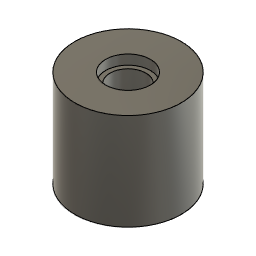
Gehaeuse (Autodesk Fusion 360 archive; units mm, degrees)
design "Befestigungsrohr"
Autodesk Fusion 360 part; units mm, degrees
sketch "Skizze1" plane through (0, 0, 0) normal (0, 1, 0) x (1, 0, 0)
sketch "Skizze2" plane through (0, 0, 0) normal (0, 1, 0) x (1, 0, 0)
  circle A0 centre (-32.0905, 19.022) radius 2.75
  circle A1 centre (-32.0905, 19.022) radius 0.925
  dimension "d1" = 5.5
  dimension "d2" = 1.85
  constraint concentric A0 A1
  measures "d1" diameter of A0
  measures "d2" diameter of A1
extrude "Extrusion1" add sketch "Skizze2" along normal blind 5
sketch "Skizze3" plane through (0, 5, 0) normal (0, 1, 0) x (-1, 0, 0)
  circle A0 centre (32.0905, -19.022) radius 0.925
  circle A1 centre (32.0905, -19.022) radius 2.75
  circle A2 centre (32.0905, -19.022) radius 1.155
  dimension "d5" = 2.31
  constraint concentric A0 A2
  measures "d5" diameter of A2
extrude "Extrusion2" cut sketch "Skizze3" against normal blind 0.5 contours A2

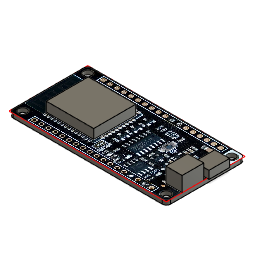
design "Microcontroller"
Autodesk Fusion 360 part; units mm, degrees
sketch "Skizze1" plane through (0, 0, 0) normal (0, 1, 0) x (1, 0, 0)
  line L0 (-42.4258, 18.0352) -> (12.5742, 18.0352)
  line L1 (14.0742, 16.5352) -> (14.0742, -9.4648)
  line L2 (12.5742, -10.9648) -> (-42.4258, -10.9648)
  line L3 (-43.9258, -9.4648) -> (-43.9258, 16.5352)
  line L4 (-14.9258, 20.3575) -> (-14.9258, -19.985) construction
  line L5 (-54.1584, 3.5352) -> (25.7033, 3.5352) construction
  circle A0 centre (-41.4258, 15.5352) radius 1.5
  circle A1 centre (11.5742, 15.5352) radius 1.5
  circle A2 centre (-41.4258, -8.4648) radius 1.5
  circle A3 centre (11.5742, -8.4648) radius 1.5
  arc A4 (-42.4258, 18.0352) -> (-43.9258, 16.5352) centre (-42.4258, 16.5352) ccw
  arc A5 (-43.9258, -9.4648) -> (-42.4258, -10.9648) centre (-42.4258, -9.4648) ccw
  arc A6 (12.5742, -10.9648) -> (14.0742, -9.4648) centre (12.5742, -9.4648) ccw
  arc A7 (14.0742, 16.5352) -> (12.5742, 18.0352) centre (12.5742, 16.5352) ccw
  line L6 (-36.7258, 11.0352) -> (-19.2258, 11.0352)
  line L7 (-19.2258, 11.0352) -> (-19.2258, -4.4648)
  line L8 (-19.2258, -4.4648) -> (-36.7258, -4.4648)
  line L9 (-36.7258, -4.4648) -> (-36.7258, 11.0352)
  line L10 (14.7742, 11.6352) -> (9.2742, 11.6352)
  line L11 (9.2742, 11.6352) -> (9.2742, 4.0352)
  line L12 (9.2742, 4.0352) -> (14.7742, 4.0352)
  line L13 (14.7742, 4.0352) -> (14.7742, 11.6352)
  line L14 (8.0742, 2.8352) -> (14.0742, 2.8352)
  line L15 (14.0742, 2.8352) -> (14.0742, -5.1648)
  line L16 (14.0742, -5.1648) -> (8.0742, -5.1648)
  line L17 (8.0742, -5.1648) -> (8.0742, 2.8352)
  point P0 (-43.9258, 18.0352)
  point P1 (14.0742, 18.0352)
  point P2 (-43.9258, -10.9648)
  dimension "d1" = 58
  dimension "d2" = 29
  dimension "d3" = 3
  dimension "d4" = 26.5
  dimension "d5" = 12
  dimension "d6" = 1.5
  dimension "d9" = 17.5
  dimension "d10" = 15.5
  dimension "d11" = 6.5
  dimension "d12" = 7.2
  dimension "d15" = 5.5
  dimension "d16" = 7.6
  dimension "d17" = 0.7
  dimension "d18" = 6.4
  dimension "d23" = 8
  dimension "d24" = 6
  dimension "d26" = 5.8
  constraint horizontal L0
  constraint vertical L1
  constraint horizontal L2
  constraint vertical L3
  constraint perpendicular L2 L4
  constraint symmetric L1 L3 L4
  constraint perpendicular L3 L5
  constraint symmetric L0 L2 L5
  constraint symmetric L4 A0 A1
  constraint symmetric L5 A0 A2
  constraint symmetric L5 A1 A3
  constraint coincident P0 L0
  constraint coincident P0 L3
  constraint tangent L0 A4
  constraint tangent L3 A4
  constraint coincident P2 L2
  constraint coincident P2 L3
  constraint tangent L2 A5
  constraint tangent L3 A5
  constraint equal A4 A5
  constraint tangent L1 A6
  constraint tangent L2 A6
  constraint equal A4 A6
  constraint coincident P1 L0
  constraint coincident P1 L1
  constraint tangent L0 A7
  constraint tangent L1 A7
  constraint equal A4 A7
  constraint horizontal L6
  constraint vertical L7
  constraint horizontal L8
  constraint vertical L9
  constraint horizontal L10
  constraint vertical L11
  constraint horizontal L12
  constraint vertical L13
  constraint horizontal L14
  constraint vertical L15
  constraint horizontal L16
  constraint vertical L17
  constraint coincident L1 L15.end
  measures "d1" distance of P0 P1
  measures "d2" distance of P0 P2
  measures "d3" diameter of A0
  measures "d4" distance of L4 A0.centre
  measures "d5" distance of L5 A0.centre
  measures "d6" radius of A4
  measures "d9" distance of L7.end L8.end
  measures "d10" distance of L6.end L7.end
  measures "d11" distance of L2 L8
  measures "d12" distance of L3 L9
  measures "d15" distance of L10.start L10.end
  measures "d16" distance of L10.end L11.end
  measures "d17" distance of L1 L13
  measures "d18" distance of L0 L10
  measures "d23" distance of L14.start L16.end
  measures "d24" distance of L14.start L14.end
  measures "d26" distance of L2 L16
extrude "Extrusion1" add sketch "Skizze1" along normal blind 1.5 contours L0 L1 L2 L3 A4 A5 A6 A7 L10 L11 L12 L14 L16 L17 | L1 L10 L11 L12 | L1 L14 L15 L16 L17 | L6 L7 L8 L9
extrude "Extrusion2" add sketch "Skizze1" along normal blind 5 contours L6 L7 L8 L9
extrude "Extrusion3" add sketch "Skizze1" along normal blind 4.4 and the other way blind -1.5 contours L1 L10 L12 L13 | L1 L10 L11 L12
extrude "Extrusion4" add sketch "Skizze1" along normal blind 7 contours L1 L14 L15 L16 L17
equation "d4 = ( 53 / 2 ) * 1 mm"
equation "d5 = ( 24 / 2 ) * 1 mm"

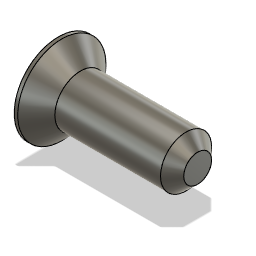
design "Schraube"
Autodesk Fusion 360 part; units mm, degrees
sketch "Skizze1" plane through (0, 0, 0) normal (0, 1, 0) x (1, 0, 0)
  line L0 (-39.2641, 12.0215) -> (10.8095, 12.0215) construction
  line L1 (-30.9471, 12.0215) -> (-30.9471, 13.9215)
  line L2 (-30.9471, 13.9215) -> (-30.7971, 13.9215)
  line L3 (-30.7971, 13.9215) -> (-29.9971, 13.1215)
  line L4 (-29.9971, 13.1215) -> (-24.9471, 13.1215)
  line L5 (-24.9471, 13.1215) -> (-24.9471, 12.0215)
  line L6 (-30.9471, 12.0215) -> (-24.9471, 12.0215)
  dimension "d1" = 135
  dimension "d2" = 6
  dimension "d3" = 1.1
  dimension "d4" = 1.9
  dimension "d5" = 0.15
  constraint horizontal L0
  constraint coincident L0 L1.start
  constraint perpendicular L0 L1
  constraint perpendicular L1 L2
  constraint perpendicular L1 L4
  constraint coincident L0 L5.end
  constraint perpendicular L0 L5
  measures "d1" angle of L3 L4
  measures "d2" distance of L1 L5
  measures "d3" distance of L4 L5.end
  measures "d4" distance of L0 L2
  measures "d5" distance of L1.end L2.end
revolve "Drehen1" add sketch "Skizze1" angle 360 about axis through (-39.2641, 0, -12.0215) along (1, 0, 0)
chamfer "Fase1" distance 0.5 angle 45 1 edges at (-24.9471, -0.3978, -10.9959)
sketch "Skizze2" plane through (-30.9471, 0, 0) normal (-1, 0, 0) x (0, 0, 1)
  circle A0 centre (-12.0215, 0) radius 1.9
  circle A1 centre (-12.0215, 0) radius 0.875
  dimension "d8" = 1.75
  constraint concentric A0 A1
  measures "d8" diameter of A1
extrude "Extrusion1" cut sketch "Skizze2" against normal blind 0.8 contours A1
equation "d4 = ( 3.8 / 2 ) * 1 mm"

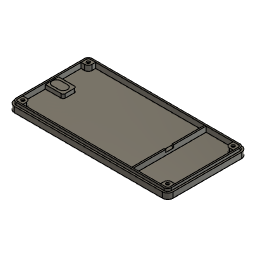
design "Gehäuseboden"
Autodesk Fusion 360 part; units mm, degrees
sketch "Skizze1" plane through (0, 0, 0) normal (0, 1, 0) x (1, 0, 0)
  line L0 (-57.1853, 33.6695) -> (54.8147, 33.6695)
  line L1 (58.8147, 29.6695) -> (58.8147, -22.3305)
  line L2 (54.8147, -26.3305) -> (-57.1853, -26.3305)
  line L3 (-61.1853, -22.3305) -> (-61.1853, 29.6695)
  arc A0 (-57.1853, 33.6695) -> (-61.1853, 29.6695) centre (-57.1853, 29.6695) ccw
  arc A1 (-61.1853, -22.3305) -> (-57.1853, -26.3305) centre (-57.1853, -22.3305) ccw
  arc A2 (54.8147, -26.3305) -> (58.8147, -22.3305) centre (54.8147, -22.3305) ccw
  arc A3 (58.8147, 29.6695) -> (54.8147, 33.6695) centre (54.8147, 29.6695) ccw
  point P0 (-61.1853, 33.6695)
  point P1 (58.8147, 33.6695)
  point P2 (-61.1853, -26.3305)
  dimension "d1" = 120
  dimension "d2" = 60
  dimension "d3" = 4
  constraint horizontal L0
  constraint vertical L1
  constraint horizontal L2
  constraint vertical L3
  constraint coincident P0 L0
  constraint coincident P0 L3
  constraint tangent L0 A0
  constraint tangent L3 A0
  constraint coincident P2 L2
  constraint coincident P2 L3
  constraint tangent L2 A1
  constraint tangent L3 A1
  constraint equal A0 A1
  constraint tangent L1 A2
  constraint tangent L2 A2
  constraint equal A0 A2
  constraint coincident P1 L0
  constraint coincident P1 L1
  constraint tangent L0 A3
  constraint tangent L1 A3
  constraint equal A0 A3
  measures "d1" distance of P0 P1
  measures "d2" distance of P0 P2
  measures "d3" radius of A0
extrude "Extrusion1" add sketch "Skizze1" against normal blind 2.5 makes body 1
ref_plane "Arbeitsebene1" through (-1.1853, -1.25, -3.6695) normal (1, 0, 0) x (0, 0, 1)
sketch "Skizze4" plane through (-1.1853, -1.25, -3.6695) normal (1, 0, 0) x (0, 0, -1)
  line L0 (-27.5, 5.25) -> (-28.65, 5.25)
  line L1 (-28.65, 5.25) -> (-28.65, 3.25)
  line L2 (-28.65, 3.25) -> (-30, 3.25)
  line L3 (-30, 3.25) -> (-30, 1.25)
  line L4 (-30, 1.25) -> (-27.5, 1.25)
  line L5 (-27.5, 5.25) -> (-27.5, 1.25)
  line L6 (26, 1.25) -> (-26, 1.25)
  dimension "d16" = 1.5
  dimension "d17" = 2.5
  dimension "d18" = 1.15
  dimension "d28" = 4
  dimension "d29" = 2
  constraint horizontal L0
  constraint perpendicular L0 L1
  constraint perpendicular L1 L2
  constraint perpendicular L2 L3
  constraint perpendicular L3 L4
  constraint perpendicular L4 L5
  constraint collinear L4 L6
  measures "d16" distance of L5 L6.end
  measures "d17" distance of L3.end L4.end
  measures "d18" distance of L0.start L0.end
  measures "d28" distance of L0.start L4.end
  measures "d29" distance of L0.end L1.end
sweep "Sweeping1" add profiles "Skizze4" along 8 edges at (-60.0137, 0, 25.1589) (-61.1853, 0, -3.6695) (-60.0137, 0, -32.4979) (-1.1853, 0, -33.6695) (57.6431, 0, -32.4979) (58.8147, 0, -3.6695) (57.6431, 0, 25.1589) (-1.1853, 0, 26.3305) section 1 on bodies 1 bodies 1
ref_plane "Arbeitsebene2" through (-1.1853, -0.25, -3.6695) normal (0, 0, 1) x (-1, 0, 0)
sketch "Skizze5" plane through (-1.1853, -0.25, -3.6695) normal (0, 0, 1) x (1, 0, 0)
  line L0 (29, 0.25, -27.5) -> (31.5, 0.25, -27.5)
  line L1 (31.5, 0.25, -27.5) -> (31.5, 4.25, -27.5)
  line L2 (31.5, 4.25, -27.5) -> (30.35, 4.25, -27.5)
  line L3 (30.35, 4.25, -27.5) -> (30.35, 2.25, -27.5)
  line L4 (30.35, 2.25, -27.5) -> (29, 2.25, -27.5)
  line L5 (29, 2.25, -27.5) -> (29, 0.25, -27.5)
  line L6 (56, 0.25, -27.5) -> (-56, 0.25, -27.5)
  line L7 (56, 4.25, -27.5) -> (56, 0.25, -27.5)
  dimension "d35" = 2.5
  dimension "d36" = 4
  dimension "d37" = 2
  dimension "d38" = 1.15
  dimension "d39" = 24.5
extrude "Extrusion2" add sketch "Skizze5" along normal up to near side of body 1 separate body contours L0 L1 L2 L3 L4 L5 L6 in plane through (-1.1853, -0.25, -31.1695) normal (0, 0, 1) makes body 2
sketch "Skizze6" plane through (30.3147, 0, 0) normal (1, 0, 0) x (0, 0, -1)
  line L0 (-23.8305, 4) -> (-23.8305, 0)
  line L1 (-23.8305, 0) -> (31.1695, 0)
  line L2 (31.1695, 0) -> (31.1695, 4)
  line L3 (31.1695, 4) -> (-23.8305, 4)
sketch "Skizze7" plane through (30.3147, 2, -3.6695) normal (1, 0, 0) x (0, 0, -1)
  line L0 (3, 2) -> (3, 0)
  line L1 (3, 0) -> (-3, 0)
  line L2 (-3, 0) -> (-3, 2)
  line L3 (27.5, 2) -> (-27.5, 2)
  line L4 (27.5, -2) -> (27.5, 2)
  line L5 (-27.5, 2) -> (-27.5, -2)
  line L6 (-3, 2) -> (3, 2)
  dimension "d42" = 6
  dimension "d43" = 2
  dimension "d44" = 24.5
  dimension "d45" = 24
  constraint vertical L0
  constraint perpendicular L0 L1
  constraint perpendicular L1 L2
  constraint coincident L3 L2.end
  constraint coincident L3 L0.start
  measures "d42" distance of L0.end L1.end
  measures "d43" distance of L1 L3
  measures "d44" distance of L0 L4
extrude "Extrusion3" cut sketch "Skizze7" against normal blind 3 bodies 2
chamfer "Fase1" distance 0.3 angle 45 1 faces at (17.4814, -2.5, 6.3305) on bodies 1
sketch "Skizze8" plane through (0, 0, 0) normal (0, 1, 0) x (-1, 0, 0)
  arc A0 (-54.8147, 23.8305) -> (-56.3147, 22.3305) centre (-54.8147, 22.3305) ccw
  line L0 (-56.3147, 22.3305) -> (-56.3147, -29.6695)
  arc A1 (-56.3147, -29.6695) -> (-54.8147, -31.1695) centre (-54.8147, -29.6695) ccw
  line L1 (-54.8147, -31.1695) -> (57.1853, -31.1695)
  arc A2 (57.1853, -31.1695) -> (58.6853, -29.6695) centre (57.1853, -29.6695) ccw
  line L2 (58.6853, -29.6695) -> (58.6853, 22.3305)
  arc A3 (58.6853, 22.3305) -> (57.1853, 23.8305) centre (57.1853, 22.3305) ccw
  line L3 (57.1853, 23.8305) -> (-54.8147, 23.8305)
  line L4 (58.6853, 18.3305) -> (55.9353, 18.3305)
  line L5 (53.1853, 21.0805) -> (53.1853, 23.8305)
  line L6 (53.1853, 23.8305) -> (58.6853, 23.8305)
  line L7 (58.6853, 23.8305) -> (58.6853, 18.3305)
  arc A4 (53.1853, 21.0805) -> (55.9353, 18.3305) centre (55.9353, 21.0805) ccw
  line L8 (-50.8147, -31.1695) -> (-56.3147, -31.1695)
  line L9 (-56.3147, -31.1695) -> (-56.3147, -25.6695)
  line L10 (-56.3147, -25.6695) -> (-53.5647, -25.6695)
  line L11 (-50.8147, -28.4195) -> (-50.8147, -31.1695)
  arc A5 (-50.8147, -28.4195) -> (-53.5647, -25.6695) centre (-53.5647, -28.4195) ccw
  point P0 (53.1853, 18.3305)
  point P1 (-50.8147, -25.6695)
  dimension "d49" = 5.5
  dimension "d50" = 5.5
  dimension "d51" = 2.75
  dimension "d52" = 5.5
  dimension "d53" = 5.5
  dimension "d54" = 2.75
  constraint horizontal L4
  constraint vertical L5
  constraint horizontal L6
  constraint vertical L7
  constraint coincident L3 L5.end
  constraint coincident L2 L4.start
  constraint coincident P0 L4
  constraint coincident P0 L5
  constraint tangent L4 A4
  constraint tangent L5 A4
  constraint horizontal L8
  constraint vertical L9
  constraint horizontal L10
  constraint vertical L11
  constraint coincident L0 L9.end
  constraint coincident L1 L8.start
  constraint coincident P1 L10
  constraint coincident P1 L11
  constraint tangent L10 A5
  constraint tangent L11 A5
  measures "d49" distance of L4.start P0
  measures "d50" distance of P0 L5.end
  measures "d51" radius of A4
  measures "d52" distance of L9.end P1
  measures "d53" distance of L8.start P1
  measures "d54" radius of A5
extrude "Extrusion4" add sketch "Skizze8" along normal up to surface (4 mm away) separate body contours L2 A3 L3 L4 L5 L6 L7 A4 | L0 A1 L1 L8 L9 L10 L11 A5 makes body 3 at (-55.9353, 0, 20.5805) makes body 4 at (53.0647, 0, -28.4195)
sketch "Skizze9" plane through (0, 4, 0) normal (0, 1, 0) x (-1, 0, 0)
  line L0 (57.1853, 23.8305) -> (53.1853, 23.8305)
  line L1 (53.1853, 23.8305) -> (53.1853, 21.0805)
  arc A0 (53.1853, 21.0805) -> (55.9353, 18.3305) centre (55.9353, 21.0805) ccw
  line L2 (55.9353, 18.3305) -> (58.6853, 18.3305)
  line L3 (58.6853, 18.3305) -> (58.6853, 22.3305)
  arc A1 (58.6853, 22.3305) -> (57.1853, 23.8305) centre (57.1853, 22.3305) ccw
  circle A2 centre (55.9353, 21.0805) radius 1.225
  circle A3 centre (-53.5647, -28.4195) radius 1.225
  line L4 (-50.8147, -28.4195) -> (-50.8147, -31.1695)
  point P0 (-53.5647, -25.6695)
  dimension "d57" = 2.45
  dimension "d58" = 2.45
  dimension "d59" = 2.75
  dimension "d60" = 2.75
  constraint concentric A0 A2
  measures "d57" diameter of A2
  measures "d58" diameter of A3
  measures "d59" distance of A3.centre L4
  measures "d60" distance of A3.centre P0
extrude "Extrusion5" cut sketch "Skizze9" against normal up to surface (6.5 mm away) contours A2 | A3 bodies 1 3 4
sketch "Skizze10" plane through (0, -2.5, 0) normal (0, -1, 0) x (1, 0, 0)
  circle A0 centre (-55.9353, 21.0805) radius 1.225
  circle A1 centre (53.5647, -28.4195) radius 1.225
  arc A2 (58.5147, 22.3305) -> (54.8147, 26.0305) centre (54.8147, 22.3305) ccw
  line L0 (54.8147, 26.0305) -> (-57.1853, 26.0305)
  arc A3 (-57.1853, 26.0305) -> (-60.8853, 22.3305) centre (-57.1853, 22.3305) ccw
  line L1 (-60.8853, 22.3305) -> (-60.8853, -29.6695)
  arc A4 (-60.8853, -29.6695) -> (-57.1853, -33.3695) centre (-57.1853, -29.6695) ccw
  line L2 (-57.1853, -33.3695) -> (54.8147, -33.3695)
  arc A5 (54.8147, -33.3695) -> (58.5147, -29.6695) centre (54.8147, -29.6695) ccw
  line L3 (58.5147, -29.6695) -> (58.5147, 22.3305)
  circle A6 centre (-55.9353, 21.0805) radius 2.25
  circle A7 centre (53.5647, -28.4195) radius 2.25
  circle A8 centre (-55.9353, -28.4195) radius 2.25
  circle A9 centre (53.5647, 21.0805) radius 2.25
  line L4 (-58.6853, 22.3305) -> (-58.6853, -29.6695)
  line L5 (-57.1853, -31.1695) -> (54.8147, -31.1695)
  line L6 (56.3147, -29.6695) -> (56.3147, 22.3305)
  line L7 (54.8147, 23.8305) -> (-57.1853, 23.8305)
  dimension "d63" = 4.5
  dimension "d64" = 4.5
  dimension "d93" = 4.5
  dimension "d94" = 4.5
  dimension "d95" = 2.75
  dimension "d96" = 2.75
  dimension "d97" = 2.75
  dimension "d98" = 2.75
  constraint concentric A0 A6
  constraint concentric A1 A7
  measures "d63" diameter of A6
  measures "d64" diameter of A7
  measures "d93" diameter of A8
  measures "d94" diameter of A9
  measures "d95" distance of A8.centre L4
  measures "d96" distance of A8.centre L5
  measures "d97" distance of A9.centre L6
  measures "d98" distance of A9.centre L7
extrude "Extrusion6" cut sketch "Skizze10" against normal blind 4.5 contours A6 | A7 bodies 1 3 4
chamfer "Fase2" distance 1 angle 45 2 edges at (-54.7932, 2, 21.5235) (54.7068, 2, -27.9765) on bodies 3 4
chamfer "Fase3" distance 0.15 angle 45 2 edges at (-58.0331, -2.5, 21.8941) (51.4669, -2.5, -27.6059) on bodies 1
sketch "Skizze11" plane through (0, 0, 0) normal (0, 1, 0) x (-1, 0, 0)
  circle A0 centre (55.9353, 21.0805) radius 2.25
  circle A1 centre (-53.5647, -28.4195) radius 2.25
  arc A2 (-54.8147, 23.8305) -> (-56.3147, 22.3305) centre (-54.8147, 22.3305) ccw
  line L0 (-56.3147, 22.3305) -> (-56.3147, -29.6695)
  arc A3 (-56.3147, -29.6695) -> (-54.8147, -31.1695) centre (-54.8147, -29.6695) ccw
  line L1 (-54.8147, -31.1695) -> (57.1853, -31.1695)
  arc A4 (57.1853, -31.1695) -> (58.6853, -29.6695) centre (57.1853, -29.6695) ccw
  line L2 (58.6853, -29.6695) -> (58.6853, 22.3305)
  arc A5 (58.6853, 22.3305) -> (57.1853, 23.8305) centre (57.1853, 22.3305) ccw
  line L3 (57.1853, 23.8305) -> (-54.8147, 23.8305)
  line L4 (55.1853, -5.4195) -> (52.9239, -5.4195)
  line L5 (55.1853, -1.9195) -> (52.9239, -1.9195)
  arc A6 (55.1853, -5.4195) -> (55.1853, -1.9195) centre (55.1853, -3.6695) ccw
  arc A7 (52.9239, -1.9195) -> (52.9239, -5.4195) centre (50.1853, -3.6695) ccw
  line L6 (58.6853, 1.3305) -> (45.1853, 1.3305)
  line L7 (45.1853, 1.3305) -> (45.1853, -8.6695)
  line L8 (45.1853, -8.6695) -> (58.6853, -8.6695)
  line L9 (58.6853, -8.6695) -> (58.6853, 1.3305)
  circle A8 centre (55.1853, -3.6695) radius 3.25
  line L10 (50.1853, -0.4195) -> (55.1853, -0.4195)
  line L11 (55.1853, -6.9195) -> (50.1853, -6.9195)
  dimension "d69" = 6.5
  dimension "d70" = 27.5
  dimension "d71" = 8.5
  dimension "d72" = 3.5
  dimension "d73" = 27.5
  dimension "d74" = 3.5
  dimension "d79" = 10
  dimension "d80" = 13.5
  dimension "d81" = 22.5
  dimension "d82" = 6.5
  constraint tangent L4 A6
  constraint horizontal L4
  constraint tangent L5 A6
  constraint horizontal L5
  constraint horizontal L6
  constraint vertical L7
  constraint horizontal L8
  constraint vertical L9
  constraint coincident L2 L6.start
  constraint concentric A6 A8
  constraint coincident A7 L10.start
  constraint coincident A8 L10.end
  constraint tangent A8 L10
  constraint parallel L5 L10
  constraint coincident A8 L11.start
  constraint coincident A7 L11.end
  constraint tangent A7 L11
  constraint parallel L4 L11
  measures "d69" diameter of A7
  measures "d70" distance of L1 A7.centre
  measures "d71" distance of L2 A7.centre
  measures "d72" diameter of A6
  measures "d73" distance of L1 A6.centre
  measures "d74" distance of L2 A6.centre
  measures "d79" distance of L6.end L7.end
  measures "d80" distance of L7.end L8.end
  measures "d81" distance of L3 L6
  measures "d82" diameter of A8
extrude "Extrusion7" cut sketch "Skizze11" against normal blind 16 contours L4 L5 A6 A7 A8 | A7 A8 picked at (53.6777, -4.2528) bodies 1
chamfer "Fase4" distance 1.5 angle 45 3 edges at (-54.0546, 0, -5.4195) (-54.0546, 0, -1.9195) (-56.9353, 0, -3.6695) on bodies 1
chamfer "Fase5" distance 0.15 angle 45 4 edges at (-46.9353, -2.5, -3.6695) (-54.0546, -2.5, -1.9195) (-54.0546, -2.5, -5.4195) (-56.9353, -2.5, -3.6695) on bodies 1
extrude "Extrusion8" add sketch "Skizze11" along normal blind 3 separate body contours L2 L6 L7 L8 L9 makes body 5
extrude "Extrusion9" add sketch "Skizze11" along normal blind 3 and the other way blind -2 separate body contours L4 L5 A6 A7 A8 | L4 L5 A6 A7 A8 | A7 A8 L11 | A7 A8 | A7 A8 L10 makes body 6
fillet "Abrundung2" radius 1.5 2 edges at (-45.1853, 1.5, -8.6695) (-45.1853, 1.5, 1.3305) on bodies 5
copy_body "Körper kopieren/einfügen1" bodies 3 makes body 7
move_body "Verschieben1" bodies 7 to x (1, 0, 0) y (0, 1, 0) z (0, 0, 1) at (0, 0, -39)
move_body "Verschieben2" bodies 7 to x (0, 0, -1) y (0, 1, 0) z (1, 0, 0) at (-35.2658, 0, -71.1048)
move_body "Verschieben3" bodies 7 to x (-1, 0, 0) y (0, 1, 0) z (0, 0, -1) at (-111.8706, 0, -35.839)
move_body "Verschieben4" bodies 7 to x (1, 0, 0) y (0, 1, 0) z (0, 0, 1) at (2.75, 0, -7.75)
copy_body "Körper kopieren/einfügen2" bodies 4 makes body 8
move_body "Verschieben5" bodies 8 to x (0, 0, 1) y (0, 1, 0) z (-1, 0, 0) at (19.6452, 0, -35.9842)
move_body "Verschieben6" bodies 8 to x (1, 0, 0) y (0, 1, 0) z (0, 0, 1) at (5.5, 0, 3.5)
extrude "Extrusion10" cut sketch "Skizze10" against normal blind 2.5 contours A8 | A9 bodies 1
chamfer "Fase6" distance 0.15 angle 45 2 edges at (51.4669, -2.5, 21.8941) (-58.0331, -2.5, -27.6059) on bodies 1
fillet "Abrundung1" [suppressed]
equation "d3 = gehauseradius"
equation "d16 = gehauseradius - 2.5 mm"
equation "d17 = dicke"
equation "d18 = dicke / 2 - ( spalt / 2 )"
equation "hoehe = 4 mm"
equation "d28 = hoehe"
equation "d29 = ueberlappung"
equation "gehauseradius = 4 mm"
equation "spalt = 0.2 mm"
equation "dicke = 2.5 mm"
equation "ueberlappung = 2 mm"
equation "sensorraum = 26 mm"
equation "d35 = dicke"
equation "d36 = hoehe"
equation "d37 = ueberlappung"
equation "d38 = dicke / 2 - spalt / 2"
equation "d39 = sensorraum - gehauseradius + dicke"

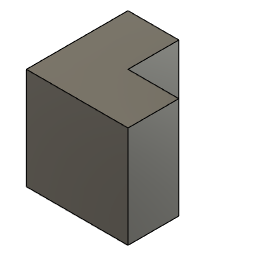
design "Ecke"
Autodesk Fusion 360 part; units mm, degrees
sketch "Skizze1" plane through (0, 0, 0) normal (0, 1, 0) x (1, 0, 0)
  line L0 (-16.0362, 31.617) -> (-13.5362, 31.617)
  line L1 (-11.0362, 29.117) -> (-11.0362, 26.617)
  line L2 (-11.0362, 26.617) -> (-16.0362, 26.617)
  line L3 (-16.0362, 26.617) -> (-16.0362, 31.617)
  line L4 (-13.5362, 31.617) -> (-13.5362, 29.117)
  line L5 (-13.5362, 29.117) -> (-11.0362, 29.117)
  dimension "d1" = 5
  dimension "d2" = 5
  constraint horizontal L0
  constraint vertical L1
  constraint horizontal L2
  constraint vertical L3
  constraint perpendicular L0 L4
  constraint perpendicular L1 L5
  measures "d1" distance of L0.start L2.end
  measures "d2" distance of L1.end L2.end
extrude "Extrusion1" add sketch "Skizze1" along normal blind 5

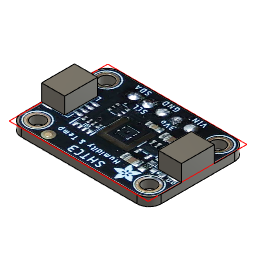
design "Sensor"
Autodesk Fusion 360 part; units mm, degrees
sketch "Skizze1" plane through (0, 0, 0) normal (0, 1, 0) x (1, 0, 0)
  line L0 (-39.1615, 29.7198) -> (-18.0615, 29.7198)
  line L1 (-15.8615, 27.5198) -> (-15.8615, 14.1198)
  line L2 (-18.0615, 11.9198) -> (-39.1615, 11.9198)
  line L3 (-41.3615, 14.1198) -> (-41.3615, 27.5198)
  line L4 (-46.6299, 20.8198) -> (-7.189, 20.8198) construction
  line L5 (-28.6115, 31.5759) -> (-28.6115, 6.919) construction
  circle A0 centre (-38.7615, 27.0698) radius 1.25
  circle A1 centre (-38.7615, 14.5698) radius 1.25
  circle A2 centre (-18.4615, 27.0698) radius 1.25
  circle A3 centre (-18.4615, 14.5698) radius 1.25
  arc A4 (-39.1615, 29.7198) -> (-41.3615, 27.5198) centre (-39.1615, 27.5198) ccw
  arc A5 (-41.3615, 14.1198) -> (-39.1615, 11.9198) centre (-39.1615, 14.1198) ccw
  arc A6 (-18.0615, 11.9198) -> (-15.8615, 14.1198) centre (-18.0615, 14.1198) ccw
  arc A7 (-15.8615, 27.5198) -> (-18.0615, 29.7198) centre (-18.0615, 27.5198) ccw
  line L6 (-41.3615, 23.8198) -> (-37.1615, 23.8198)
  line L7 (-37.1615, 23.8198) -> (-37.1615, 17.8198)
  line L8 (-37.1615, 17.8198) -> (-41.3615, 17.8198)
  line L9 (-41.3615, 17.8198) -> (-41.3615, 23.8198)
  line L10 (-20.0615, 17.8198) -> (-15.8615, 17.8198)
  line L11 (-20.0615, 23.8198) -> (-20.0615, 17.8198)
  line L12 (-15.8615, 23.8198) -> (-20.0615, 23.8198)
  line L13 (-15.8615, 17.8198) -> (-15.8615, 23.8198)
  point P0 (-41.3615, 29.7198)
  point P1 (-15.8615, 29.7198)
  point P2 (-41.3615, 11.9198)
  dimension "d1" = 25.5
  dimension "d2" = 17.8
  dimension "d3" = 2.5
  dimension "d4" = 10.15
  dimension "d5" = 6.25
  dimension "d6" = 2.2
  dimension "d7" = 2.2
  dimension "d8" = 4.2
  dimension "d9" = 6
  dimension "d10" = 3
  constraint horizontal L0
  constraint vertical L1
  constraint horizontal L2
  constraint vertical L3
  constraint horizontal L4
  constraint perpendicular L4 L5
  constraint symmetric L0 L2 L4
  constraint symmetric L1 L3 L5
  constraint symmetric L4 A0 A1
  constraint symmetric L5 A0 A2
  constraint symmetric L5 A1 A3
  constraint coincident P0 L0
  constraint coincident P0 L3
  constraint tangent L0 A4
  constraint tangent L3 A4
  constraint coincident P2 L2
  constraint coincident P2 L3
  constraint tangent L2 A5
  constraint tangent L3 A5
  constraint tangent L1 A6
  constraint tangent L2 A6
  constraint equal A5 A6
  constraint coincident P1 L0
  constraint coincident P1 L1
  constraint tangent L0 A7
  constraint tangent L1 A7
  constraint equal A5 A7
  constraint horizontal L6
  constraint vertical L7
  constraint horizontal L8
  constraint vertical L9
  constraint coincident L3 L6.start
  constraint symmetric L5 L6.start L12.start
  constraint symmetric L5 L6.end L11.start
  constraint symmetric L5 L7.end L10.start
  constraint symmetric L5 L8.end L10.end
  measures "d1" distance of P0 P1
  measures "d2" distance of P0 P2
  measures "d3" diameter of A0
  measures "d4" distance of L5 A0.centre
  measures "d5" distance of L4 A0.centre
  measures "d6" radius of A4
  measures "d7" radius of A5
  measures "d8" distance of L6.start L6.end
  measures "d9" distance of L6.end L7.end
  measures "d10" distance of L4 L6
extrude "Extrusion1" add sketch "Skizze1" along normal blind 1.5 contours L0 L1 L2 L3 A4 A5 A6 A7 L6 L7 L8 L10 L11 L12
extrude "Extrusion2" add sketch "Skizze1" along normal blind 4.5 contours L3 L6 L7 L8 L9 | L1 L10 L11 L12 L13
equation "d4 = ( 20.3 / 2 ) * 1 mm"
equation "d5 = ( 12.5 / 2 ) * 1 mm"

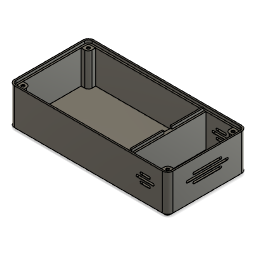
design "Gehäusedeckel"
Autodesk Fusion 360 part; units mm, degrees
sketch "Skizze1" plane through (0, 0, 0) normal (0, 1, 0) x (1, 0, 0)
  line L0 (-57.1853, 33.6695) -> (54.8147, 33.6695)
  line L1 (58.8147, 29.6695) -> (58.8147, -22.3305)
  line L2 (54.8147, -26.3305) -> (-57.1853, -26.3305)
  line L3 (-61.1853, -22.3305) -> (-61.1853, 29.6695)
  arc A0 (-57.1853, 33.6695) -> (-61.1853, 29.6695) centre (-57.1853, 29.6695) ccw
  arc A1 (-61.1853, -22.3305) -> (-57.1853, -26.3305) centre (-57.1853, -22.3305) ccw
  arc A2 (54.8147, -26.3305) -> (58.8147, -22.3305) centre (54.8147, -22.3305) ccw
  arc A3 (58.8147, 29.6695) -> (54.8147, 33.6695) centre (54.8147, 29.6695) ccw
  point P0 (-61.1853, 33.6695)
  point P1 (58.8147, 33.6695)
  point P2 (-61.1853, -26.3305)
  dimension "d1" = 120
  dimension "d2" = 60
  dimension "d3" = 4
  constraint horizontal L0
  constraint vertical L1
  constraint horizontal L2
  constraint vertical L3
  constraint coincident P0 L0
  constraint coincident P0 L3
  constraint tangent L0 A0
  constraint tangent L3 A0
  constraint coincident P2 L2
  constraint coincident P2 L3
  constraint tangent L2 A1
  constraint tangent L3 A1
  constraint equal A0 A1
  constraint tangent L1 A2
  constraint tangent L2 A2
  constraint equal A0 A2
  constraint coincident P1 L0
  constraint coincident P1 L1
  constraint tangent L0 A3
  constraint tangent L1 A3
  constraint equal A0 A3
  measures "d1" distance of P0 P1
  measures "d2" distance of P0 P2
  measures "d3" radius of A0
extrude "Extrusion1" add sketch "Skizze1" against normal blind 2.5 makes body 1
ref_plane "Arbeitsebene1" through (-1.1853, -1.25, -3.6695) normal (1, 0, 0) x (0, 0, 1)
sketch "Skizze4" plane through (-1.1853, -1.25, -3.6695) normal (1, 0, 0) x (0, 0, -1)
  line L0 (-30, 28.25) -> (-30, 1.25)
  line L1 (-30, 1.25) -> (-27.5, 1.25)
  line L2 (-27.5, 26.25) -> (-27.5, 1.25)
  line L3 (26, 1.25) -> (-26, 1.25)
  line L4 (-30, 28.25) -> (-28.85, 28.25)
  line L5 (-28.85, 28.25) -> (-28.85, 26.25)
  line L6 (-27.5, 26.25) -> (-28.85, 26.25)
  dimension "d16" = 1.5
  dimension "d17" = 2.5
  dimension "d48" = 27
  dimension "d49" = 2
  dimension "d50" = 1.15
  constraint perpendicular L0 L1
  constraint perpendicular L1 L2
  constraint collinear L1 L3
  constraint perpendicular L0 L4
  constraint perpendicular L4 L5
  constraint perpendicular L5 L6
  measures "d16" distance of L2 L3.end
  measures "d17" distance of L0.end L1.end
  measures "d48" distance of L0.start L0.end
  measures "d49" distance of L4.end L5.end
  measures "d50" distance of L0.start L4.end
sweep "Sweeping1" add profiles "Skizze4" along 8 edges at (-60.0137, 0, 25.1589) (-61.1853, 0, -3.6695) (-60.0137, 0, -32.4979) (-1.1853, 0, -33.6695) (57.6431, 0, -32.4979) (58.8147, 0, -3.6695) (57.6431, 0, 25.1589) (-1.1853, 0, 26.3305) section 1 on bodies 1 bodies 1
ref_plane "Arbeitsebene2" through (-1.1853, 12.25, -3.6695) normal (0, 0, 1) x (-1, 0, 0)
sketch "Skizze8" plane through (0, 0, -31.1695) normal (0, 0, 1) x (1, 0, 0)
  line L0 (-57.1853, 25) -> (-57.1853, 0)
  line L1 (-57.1853, 0) -> (54.8147, 0)
  line L2 (54.8147, 0) -> (54.8147, 25)
  line L3 (54.8147, 25) -> (-57.1853, 25)
  line L4 (28.9647, 27) -> (27.8147, 27)
  line L5 (27.8147, 27) -> (27.8147, 0)
  line L6 (27.8147, 0) -> (30.3147, 0)
  line L7 (30.3147, 0) -> (30.3147, 25)
  line L8 (28.9647, 27) -> (28.9647, 25)
  line L9 (30.3147, 25) -> (28.9647, 25)
  dimension "d51" = 27
  dimension "d52" = 2.5
  dimension "d53" = 24.5
  dimension "d54" = 1.15
  dimension "d55" = 2
  constraint parallel L3 L4
  constraint perpendicular L3 L5
  constraint perpendicular L5 L6
  constraint coincident L3 L7.end
  constraint perpendicular L3 L7
  constraint perpendicular L3 L8
  constraint coincident L3 L8.end
  measures "d51" distance of L4.end L5.end
  measures "d52" distance of L5.end L6.end
  measures "d53" distance of L2 L7
  measures "d54" distance of L4.start L4.end
  measures "d55" distance of L4.start L8.end
extrude "Extrusion4" add sketch "Skizze8" along normal up to surface (55 mm away) separate body contours L3 L4 L5 L8 | L1 L3 L5 L6 L7 L9 makes body 2
sketch "Skizze9" plane through (0, 0, 23.8305) normal (0, 0, 1) x (1, 0, 0)
  line L0 (28.9647, 25) -> (28.9647, 27)
  line L1 (28.9647, 27) -> (27.8147, 27)
  line L2 (27.8147, 27) -> (27.8147, 0)
  line L3 (27.8147, 0) -> (30.3147, 0)
  line L4 (30.3147, 0) -> (30.3147, 25)
  line L5 (30.3147, 25) -> (28.9647, 25)
  line L6 (27.8147, 27) -> (28.9647, 27)
  line L7 (28.9647, 27) -> (28.9647, 25)
  line L8 (28.9647, 25) -> (27.8147, 25)
  line L9 (27.8147, 25) -> (27.8147, 27)
  constraint horizontal L6
  constraint vertical L7
  constraint horizontal L8
  constraint vertical L9
  constraint coincident L0.start L5.end
  constraint coincident L1.end L2.start
extrude "Extrusion5" cut sketch "Skizze9" against normal blind 0.2 contours L0 L1 L2 L6 L7 L8 L9 bodies 2
sketch "Skizze10" plane through (0, 0, -31.1695) normal (0, 0, -1) x (-1, 0, 0)
  line L0 (-27.8147, 27) -> (-28.9647, 27)
  line L1 (-28.9647, 27) -> (-28.9647, 25)
  line L2 (-28.9647, 25) -> (-30.3147, 25)
  line L3 (-30.3147, 25) -> (-30.3147, 0)
  line L4 (-30.3147, 0) -> (-27.8147, 0)
  line L5 (-27.8147, 0) -> (-27.8147, 27)
  line L6 (-28.9647, 27) -> (-27.8147, 27)
  line L7 (-27.8147, 27) -> (-27.8147, 25)
  line L8 (-27.8147, 25) -> (-28.9647, 25)
  line L9 (-28.9647, 25) -> (-28.9647, 27)
  dimension "d60" = 2
  constraint horizontal L6
  constraint vertical L7
  constraint horizontal L8
  constraint vertical L9
  constraint coincident L0.end L1.start
  measures "d60" distance of L0.end L1.end
extrude "Extrusion6" cut sketch "Skizze10" against normal blind 0.2 contours L0 L1 L5 L6 L7 L8 L9 bodies 2
sketch "Skizze11" plane through (27.8147, 0, 0) normal (-1, 0, 0) x (0, 0, 1)
  line L0 (-30.9695, 27) -> (-30.9695, 25)
  line L1 (-30.9695, 25) -> (-31.1695, 25)
  line L2 (-31.1695, 25) -> (-31.1695, 0)
  line L3 (-31.1695, 0) -> (23.8305, 0)
  line L4 (23.8305, 0) -> (23.8305, 25)
  line L5 (23.8305, 25) -> (23.6305, 25)
  line L6 (23.6305, 25) -> (23.6305, 27)
  line L7 (23.6305, 27) -> (-30.9695, 27)
  line L8 (-6.6695, 27) -> (-0.6695, 27)
  line L9 (-0.6695, 27) -> (-0.6695, 25)
  line L10 (-0.6695, 25) -> (-6.6695, 25)
  line L11 (-6.6695, 25) -> (-6.6695, 27)
  dimension "d63" = 6
  dimension "d64" = 2
  dimension "d65" = 24.5
  dimension "d66" = 24.5
  constraint horizontal L8
  constraint vertical L9
  constraint horizontal L10
  constraint vertical L11
  constraint coincident L7 L8.start
  measures "d63" distance of L9.end L10.end
  measures "d64" distance of L8.end L9.end
  measures "d65" distance of L4 L9
  measures "d66" distance of L2 L11
extrude "Extrusion7" cut sketch "Skizze11" against normal blind 4 contours L7 L8 L9 L10 L11 bodies 2
chamfer "Fase1" distance 2 angle 45 1 faces at (17.4814, -2.5, 6.3305) on bodies 1
sketch "Skizze12" plane through (0, 0, 0) normal (0, 1, 0) x (-1, 0, 0)
  arc A0 (-54.8147, 23.8305) -> (-56.3147, 22.3305) centre (-54.8147, 22.3305) ccw
  line L0 (-56.3147, 22.3305) -> (-56.3147, -29.6695)
  arc A1 (-56.3147, -29.6695) -> (-54.8147, -31.1695) centre (-54.8147, -29.6695) ccw
  line L1 (-54.8147, -31.1695) -> (57.1853, -31.1695)
  arc A2 (57.1853, -31.1695) -> (58.6853, -29.6695) centre (57.1853, -29.6695) ccw
  line L2 (58.6853, -29.6695) -> (58.6853, 22.3305)
  arc A3 (58.6853, 22.3305) -> (57.1853, 23.8305) centre (57.1853, 22.3305) ccw
  line L3 (57.1853, 23.8305) -> (-54.8147, 23.8305)
  line L4 (58.6853, -25.6695) -> (55.9353, -25.6695)
  line L5 (53.1853, -28.4195) -> (53.1853, -31.1695)
  line L6 (53.1853, -31.1695) -> (58.6853, -31.1695)
  line L7 (58.6853, -31.1695) -> (58.6853, -25.6695)
  arc A4 (55.9353, -25.6695) -> (53.1853, -28.4195) centre (55.9353, -28.4195) ccw
  line L8 (-56.3147, 18.3305) -> (-53.5647, 18.3305)
  line L9 (-50.8147, 21.0805) -> (-50.8147, 23.8305)
  line L10 (-50.8147, 23.8305) -> (-56.3147, 23.8305)
  line L11 (-56.3147, 23.8305) -> (-56.3147, 18.3305)
  arc A5 (-53.5647, 18.3305) -> (-50.8147, 21.0805) centre (-53.5647, 21.0805) ccw
  point P0 (53.1853, -25.6695)
  point P1 (-50.8147, 18.3305)
  dimension "d72" = 5.5
  dimension "d73" = 5.5
  dimension "d74" = 2.75
  dimension "d75" = 5.5
  dimension "d76" = 5.5
  dimension "d77" = 2.75
  constraint horizontal L4
  constraint vertical L5
  constraint horizontal L6
  constraint vertical L7
  constraint coincident L1 L5.end
  constraint coincident L2 L4.start
  constraint coincident P0 L4
  constraint coincident P0 L5
  constraint tangent L4 A4
  constraint tangent L5 A4
  constraint horizontal L8
  constraint vertical L9
  constraint horizontal L10
  constraint vertical L11
  constraint coincident L3 L9.end
  constraint coincident L0 L8.start
  constraint coincident P1 L8
  constraint coincident P1 L9
  constraint tangent L8 A5
  constraint tangent L9 A5
  measures "d72" distance of L4.start P0
  measures "d73" distance of P0 L5.end
  measures "d74" radius of A4
  measures "d75" distance of L8.start P1
  measures "d76" distance of P1 L9.end
  measures "d77" radius of A5
extrude "Extrusion8" add sketch "Skizze12" along normal up to surface (25 mm away) separate body contours A0 L0 L3 L8 L9 L10 L11 A5 | L1 A2 L2 L4 L5 L6 L7 A4 makes body 3 at (-54.2354, 16.6667, -26.2579) makes body 4 at (52.9163, 16.6667, 18.408)
sketch "Skizze13" plane through (0, 25, 0) normal (0, 1, 0) x (-1, 0, 0)
  line L0 (58.6853, -25.6695) -> (55.9353, -25.6695)
  arc A0 (55.9353, -25.6695) -> (53.1853, -28.4195) centre (55.9353, -28.4195) ccw
  line L1 (53.1853, -28.4195) -> (53.1853, -31.1695)
  line L2 (53.1853, -31.1695) -> (57.1853, -31.1695)
  arc A1 (57.1853, -31.1695) -> (58.6853, -29.6695) centre (57.1853, -29.6695) ccw
  line L3 (58.6853, -29.6695) -> (58.6853, -25.6695)
  circle A2 centre (55.9353, -28.4195) radius 0.925
  circle A3 centre (-53.5647, 21.0805) radius 0.925
  line L4 (-53.5647, 18.3305) -> (-56.3147, 18.3305)
  line L5 (-50.8147, 23.8305) -> (-50.8147, 21.0805)
  circle A4 centre (55.9353, -28.4195) radius 1.155
  circle A5 centre (-53.5647, 21.0805) radius 1.155
  dimension "d80" = 1.85
  dimension "d81" = 1.85
  dimension "d82" = 2.75
  dimension "d83" = 2.75
  dimension "d84" = 2.75
  dimension "d85" = 2.75
  dimension "d86" = 2.31
  dimension "d87" = 2.31
  constraint concentric A0 A2
  constraint concentric A2 A4
  constraint concentric A3 A5
  measures "d80" diameter of A2
  measures "d81" diameter of A3
  measures "d82" distance of A3.centre L4
  measures "d83" distance of A3.centre L5
  measures "d84" distance of L1 A0.centre
  measures "d85" distance of L0 A0.centre
  measures "d86" diameter of A4
  measures "d87" diameter of A5
extrude "Extrusion9" cut sketch "Skizze13" against normal blind 10 contours A2 | A3 bodies 3 4
extrude "Extrusion10" cut sketch "Skizze13" against normal blind 0.5 contours A4 | A5 bodies 3 4
sketch "Skizze14" plane through (58.8147, 0, 0) normal (1, 0, 0) x (0, 0, -1)
  line L0 (-22.3305, -0.5) -> (29.6695, -0.5)
  line L1 (29.6695, -0.5) -> (29.6695, 27)
  line L2 (29.6695, 27) -> (-22.3305, 27)
  line L3 (-22.3305, 27) -> (-22.3305, -0.5)
  line L4 (3.6695, -13) -> (3.6695, 32)
  line L5 (-6.3305, 16.75) -> (13.6695, 16.75)
  arc A0 (13.6695, 16.75) -> (13.6695, 18.25) centre (13.6695, 17.5) ccw
  line L6 (13.6695, 18.25) -> (-6.3305, 18.25)
  arc A1 (-6.3305, 18.25) -> (-6.3305, 16.75) centre (-6.3305, 17.5) ccw
  line L7 (-6.3305, 17.5) -> (13.6695, 17.5) construction
  line L8 (-11.3305, 13.75) -> (18.6695, 13.75)
  arc A2 (-11.3305, 15.25) -> (-11.3305, 13.75) centre (-11.3305, 14.5) ccw
  line L9 (-11.3305, 14.5) -> (18.6695, 14.5) construction
  arc A3 (18.6695, 13.75) -> (18.6695, 15.25) centre (18.6695, 14.5) ccw
  line L10 (18.6695, 15.25) -> (-11.3305, 15.25)
  line L11 (-6.3305, 10.75) -> (13.6695, 10.75)
  arc A4 (-6.3305, 12.25) -> (-6.3305, 10.75) centre (-6.3305, 11.5) ccw
  line L12 (-6.3305, 11.5) -> (13.6695, 11.5) construction
  arc A5 (13.6695, 10.75) -> (13.6695, 12.25) centre (13.6695, 11.5) ccw
  line L13 (13.6695, 12.25) -> (-6.3305, 12.25)
  dimension "d101" = 1.5
  dimension "d103" = 1.5
  dimension "d105" = 1.5
  dimension "d107" = 30
  dimension "d108" = 3
  dimension "d109" = 3
  dimension "d111" = 20
  dimension "d112" = 20
  dimension "d127" = 9.5
  constraint tangent L5 A0
  constraint tangent A0 L6
  constraint parallel L5 L6
  constraint tangent L6 A1
  constraint tangent L5 A1
  constraint perpendicular L4 L7
  constraint symmetric L4 A1.centre A0.centre
  constraint tangent L8 A3
  constraint tangent A3 L10
  constraint parallel L8 L10
  constraint tangent A2 L10
  constraint tangent L8 A2
  constraint tangent L11 A5
  constraint tangent A5 L13
  constraint parallel L11 L13
  constraint tangent A4 L13
  constraint tangent L11 A4
  constraint symmetric L4 L9.end A2.centre
  constraint symmetric L4 L12.end A4.centre
  measures "d101" diameter of A0
  measures "d103" diameter of A3
  measures "d105" diameter of A5
  measures "d107" distance of L9.end A2.centre
  measures "d108" distance of L7 L9
  measures "d109" vertical distance of L9.end L12.end
  measures "d111" distance of L12.end A4.centre
  measures "d112" distance of A1.centre A0.centre
  measures "d127" distance of L2 L7
extrude "Extrusion11" cut sketch "Skizze14" against normal blind 4 contours L4 L11 A4 L13 | L4 L11 A5 L13 | L4 L5 A0 L6 | L4 L5 L6 A1 | L4 L8 A2 L10 | L4 L8 A3 L10 bodies 1
sketch "Skizze15" plane through (0, 0, 26.3305) normal (0, 0, 1) x (1, 0, 0)
  line L0 (-57.1853, -0.5) -> (54.8147, -0.5)
  line L1 (54.8147, -0.5) -> (54.8147, 27)
  line L2 (54.8147, 27) -> (-57.1853, 27)
  line L3 (-57.1853, 27) -> (-57.1853, -0.5)
  line L4 (41.8147, 32.5) -> (41.8147, -13.5) construction
  line L5 (38.8147, 16.75) -> (44.8147, 16.75)
  arc A0 (44.8147, 16.75) -> (44.8147, 18.25) centre (44.8147, 17.5) ccw
  line L6 (44.8147, 18.25) -> (38.8147, 18.25)
  arc A1 (38.8147, 18.25) -> (38.8147, 16.75) centre (38.8147, 17.5) ccw
  line L7 (38.8147, 17.5) -> (44.8147, 17.5) construction
  line L8 (35.8147, 13.75) -> (47.8147, 13.75)
  arc A2 (47.8147, 13.75) -> (47.8147, 15.25) centre (47.8147, 14.5) ccw
  line L9 (47.8147, 15.25) -> (35.8147, 15.25)
  arc A3 (35.8147, 15.25) -> (35.8147, 13.75) centre (35.8147, 14.5) ccw
  line L10 (35.8147, 14.5) -> (47.8147, 14.5) construction
  line L11 (38.8147, 10.75) -> (44.8147, 10.75)
  arc A4 (44.8147, 10.75) -> (44.8147, 12.25) centre (44.8147, 11.5) ccw
  line L12 (44.8147, 12.25) -> (38.8147, 12.25)
  arc A5 (38.8147, 12.25) -> (38.8147, 10.75) centre (38.8147, 11.5) ccw
  line L13 (38.8147, 11.5) -> (44.8147, 11.5) construction
  dimension "d115" = 1.5
  dimension "d116" = 1.5
  dimension "d117" = 1.5
  dimension "d118" = 9.5
  dimension "d119" = 3
  dimension "d120" = 3
  dimension "d121" = 6
  dimension "d122" = 12
  dimension "d123" = 6
  dimension "d124" = 13
  constraint perpendicular L0 L4
  constraint tangent L5 A0
  constraint tangent A0 L6
  constraint parallel L5 L6
  constraint tangent L6 A1
  constraint tangent L5 A1
  constraint parallel L2 L7
  constraint tangent L8 A2
  constraint tangent A2 L9
  constraint parallel L8 L9
  constraint tangent L9 A3
  constraint tangent L8 A3
  constraint horizontal L10
  constraint tangent L11 A4
  constraint tangent A4 L12
  constraint parallel L11 L12
  constraint tangent L12 A5
  constraint tangent L11 A5
  constraint horizontal L13
  constraint symmetric L4 A1.centre A0.centre
  constraint symmetric L4 A3.centre A2.centre
  constraint symmetric L4 A5.centre A4.centre
  measures "d115" diameter of A0
  measures "d116" diameter of A2
  measures "d117" diameter of A4
  measures "d118" distance of L2 L7
  measures "d119" distance of L7 L10
  measures "d120" distance of L10 L13
  measures "d121" distance of A1.centre A0.centre
  measures "d122" distance of A3.centre A2.centre
  measures "d123" distance of A5.centre A4.centre
  measures "d124" distance of L1 L4
extrude "Extrusion12" cut sketch "Skizze15" against normal blind 64 contours L5 A0 L6 A1 | L8 A2 L9 A3 | L11 A4 L12 A5 bodies 1
chamfer "Fase2" distance 0.1 angle 45 36 edges at (41.8147, 10.75, -33.6695) (45.5647, 11.5, -33.6695) (41.8147, 12.25, -33.6695) (38.0647, 11.5, -33.6695) (41.8147, 13.75, -33.6695) (48.5647, 14.5, -33.6695) (41.8147, 15.25, -33.6695) (35.0647, 14.5, -33.6695) (41.8147, 18.25, -33.6695) (38.0647, 17.5, -33.6695) (41.8147, 16.75, -33.6695) (45.5647, 17.5, -33.6695) (58.8147, 10.75, -3.6695) (58.8147, 11.5, 7.0805) (58.8147, 12.25, -3.6695) (58.8147, 11.5, -14.4195) (58.8147, 13.75, -3.6695) (58.8147, 14.5, 12.0805) (58.8147, 15.25, -3.6695) (58.8147, 14.5, -19.4195) (58.8147, 16.75, -3.6695) (58.8147, 17.5, 7.0805) (58.8147, 18.25, -3.6695) (58.8147, 17.5, -14.4195) (41.8147, 10.75, 26.3305) (38.0647, 11.5, 26.3305) (41.8147, 12.25, 26.3305) (45.5647, 11.5, 26.3305) (41.8147, 13.75, 26.3305) (35.0647, 14.5, 26.3305) (41.8147, 15.25, 26.3305) (48.5647, 14.5, 26.3305) (41.8147, 16.75, 26.3305) (38.0647, 17.5, 26.3305) (41.8147, 18.25, 26.3305) (45.5647, 17.5, 26.3305) on bodies 1
chamfer "Fase3" distance 0.1 angle 45 36 edges at (41.8147, 18.25, 23.8305) (38.0647, 17.5, 23.8305) (41.8147, 16.75, 23.8305) (45.5647, 17.5, 23.8305) (41.8147, 15.25, 23.8305) (35.0647, 14.5, 23.8305) (41.8147, 13.75, 23.8305) (48.5647, 14.5, 23.8305) (41.8147, 12.25, 23.8305) (38.0647, 11.5, 23.8305) (41.8147, 10.75, 23.8305) (45.5647, 11.5, 23.8305) (56.3147, 18.25, -3.6695) (56.3147, 17.5, 7.0805) (56.3147, 16.75, -3.6695) (56.3147, 17.5, -14.4195) (56.3147, 15.25, -3.6695) (56.3147, 14.5, 12.0805) (56.3147, 13.75, -3.6695) (56.3147, 14.5, -19.4195) (56.3147, 12.25, -3.6695) (56.3147, 11.5, 7.0805) (56.3147, 10.75, -3.6695) (56.3147, 11.5, -14.4195) (41.8147, 12.25, -31.1695) (45.5647, 11.5, -31.1695) (41.8147, 10.75, -31.1695) (38.0647, 11.5, -31.1695) (41.8147, 15.25, -31.1695) (48.5647, 14.5, -31.1695) (41.8147, 13.75, -31.1695) (35.0647, 14.5, -31.1695) (41.8147, 18.25, -31.1695) (45.5647, 17.5, -31.1695) (41.8147, 16.75, -31.1695) (38.0647, 17.5, -31.1695) on bodies 1
copy_body "Körper kopieren/einfügen1" bodies 3 makes body 5
move_body "Verschieben1" bodies 5 to x (0, 0, -1) y (0, 1, 0) z (1, 0, 0) at (-27.5158, 0, -34.8548)
copy_body "Körper kopieren/einfügen2" bodies 4 makes body 6
move_body "Verschieben2" bodies 6 to x (0, 0, -1) y (0, 1, 0) z (1, 0, 0) at (32.2342, 0, 30.8952)
move_body "Verschieben3" bodies 6 to x (1, 0, 0) y (0, 1, 0) z (0, 0, 1) at (1.3107, 0, -6.8107)
move_body "Verschieben4" bodies 6 to x (1, 0, 0) y (0, 1, 0) z (0, 0, 1) at (-5, 0, 8)
move_body "Verschieben5" bodies 6 to x (1, 0, 0) y (0, 1, 0) z (0, 0, 1) at (3.9393, 0, -6.9393)
fillet "Abrundung1" [suppressed]
extrude "Extrusion2" [suppressed]
sketch "Skizze6" plane through (30.3147, 0, 0) normal (1, 0, 0) x (0, 0, -1)
  line L0 (-23.8305, 4) -> (-23.8305, 0)
  line L1 (-23.8305, 0) -> (31.1695, 0)
  line L2 (31.1695, 0) -> (31.1695, 4)
  line L3 (31.1695, 4) -> (-23.8305, 4)
sketch "Skizze7" plane through (30.3147, 2, -3.6695) normal (1, 0, 0) x (0, 0, -1)
  line L0 (3, 2) -> (3, 0)
  line L1 (3, 0) -> (-3, 0)
  line L2 (-3, 0) -> (-3, 2)
  line L3 (27.5, 2) -> (-27.5, 2)
  line L4 (27.5, -2) -> (27.5, 2)
  line L5 (-27.5, 2) -> (-27.5, -2)
  line L6 (-3, 2) -> (3, 2)
  dimension "d42" = 6
  dimension "d43" = 2
  dimension "d44" = 24.5
  dimension "d45" = 24
  constraint vertical L0
  constraint perpendicular L0 L1
  constraint perpendicular L1 L2
  constraint coincident L3 L2.end
  constraint coincident L3 L0.start
  measures "d42" distance of L0.end L1.end
  measures "d43" distance of L1 L3
  measures "d44" distance of L0 L4
extrude "Extrusion3" [suppressed]
equation "d3 = gehauseradius"
equation "d16 = gehauseradius - 2.5 mm"
equation "d17 = dicke"
equation "hoehe = 27 mm"
equation "gehauseradius = 4 mm"
equation "spalt = 0.2 mm"
equation "dicke = 2.5 mm"
equation "ueberlappung = 2 mm"
equation "sensorraum = 26 mm"
equation "d48 = hoehe"
equation "d49 = ueberlappung"
equation "d50 = dicke / 2 - spalt / 2"
equation "d51 = hoehe"
equation "d52 = dicke"
equation "d53 = sensorraum - gehauseradius + dicke"
equation "d54 = dicke / 2 - spalt / 2"
equation "d55 = ueberlappung"
